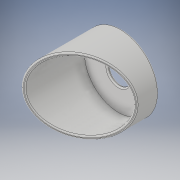
# Autodesk Inventor part: cover
Saved by Autodesk Inventor 2019 (Build 230136000, 136)
## iProperties
Created: 2024-04-30
Part Number: cover
Material: Generisch
Document SubType Name: Modeling
Designer: nic
Density: 1 g/cm^3
Appearance: Vorgabe
Author: nic
Autodesk Inventor part; units mm, degrees
ref_plane "YZ Plane" through (0, 0, 0) normal (1, 0, 0) x (0, 1, 0)
ref_plane "XZ Plane" through (0, 0, 0) normal (0, 1, 0) x (-1, 0, 0)
ref_plane "XY Plane" through (0, 0, 0) normal (0, 0, 1) x (1, 0, 0)
sketch "Skizze1" plane through (0, 0, 0) normal (0, 0, 1) x (1, 0, 0)
  circle A0 centre (0, 0) radius 52.5
  circle A1 centre (0, 0) radius 57.5
  dimension "d0" = 105
  dimension "d1" = 5
  constraints: 2 centre point, 1 coincident
  measures "d0" diameter of A0
  measures "d1" radial gap between concentric circles of A0 A1
extrude "Extrusion1" add sketch "Skizze1" along normal blind 100
sketch "Skizze2" plane through (0, 0, 0) normal (0, 0, -1) x (-1, 0, 0)
  circle A0 centre (0, 0) radius 52.5
  dimension "d15" = 105
  constraints: 1 centre point, 1 coincident
  measures "d15" diameter of A0
extrude "Extrusion2" add sketch "Skizze2" against normal blind 5
sketch "Skizze3" plane through (0, 0, 0) normal (0, 1, 0) x (-1, 0, 0)
  line L0 (57.5, 100) -> (-57.5, 100) projected
  line L1 (57.5, 100) -> (-57.5, 33.0047)
  line L2 (-57.5, 0) -> (-57.5, 100) projected
  line L3 (57.5, 100) -> (-57.5, 100)
  line L4 (-57.5, 100) -> (-57.5, 33.0047)
  constraints: 6 end point, 1 horizontal, 1 perpendicular, 1 point on line
fillet "Rundung2" radius 2 1 edges at (-57.5, 0, 0)
sketch "Skizze4" plane through (0, 0, 5) normal (0, 0, 1) x (1, 0, 0)
  circle A0 centre (0, 0) radius 17.5
  dimension "d10" = 35
  constraints: 1 centre point, 1 coincident
  measures "d10" diameter of A0
extrude "Extrusion4" cut sketch "Skizze4" against normal blind 100
fillet "Rundung3" radius 2 2 edges at (-17.5, 0, 0) (-17.5, 0, 5)
extrude "Extrusion5" cut sketch "Skizze3" along normal through all both and the other way through all
fillet "Rundung5" radius 2 3 edges at (-52.5, 0, 97.0872) (0, -57.5, 66.5024) (0, 57.5, 66.5024)
